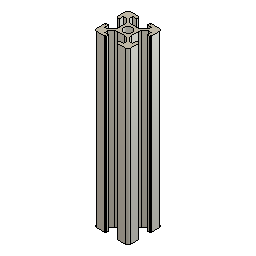
20X20 - T-slot - Aluminium Profile (Autodesk Fusion 360 design; units mm, degrees)
Autodesk Fusion 360 part; units mm, degrees
sketch "Sketch1" plane through (0, 0, 0) normal (0, 1, 0) x (1, 0, 0)
  circle A0 centre (16.6339, -3.4008) radius 2.5
  line L0 (13.0339, 6.0992) -> (13.0339, 6.5992)
  line L1 (6.6339, 0.1992) -> (7.1339, 0.1992)
  line L2 (6.6339, 0.1992) -> (7.1339, 0.1992)
  line L3 (10.0732, 2.0992) -> (8.4339, 2.0992)
  line L4 (11.1339, 4.7992) -> (11.1339, 3.1598)
  line L5 (13.5339, 4.7992) -> (13.5339, 6.0992)
  line L6 (20.2339, 6.5992) -> (20.2339, 6.0992)
  line L7 (19.7339, 6.0992) -> (19.7339, 4.7992)
  line L8 (22.1339, 4.7992) -> (19.7339, 4.7992)
  line L9 (13.5339, 4.7992) -> (11.1339, 4.7992)
  line L10 (20.2339, 6.0992) -> (19.7339, 6.0992)
  line L11 (13.5339, 6.0992) -> (13.0339, 6.0992)
  line L12 (25.1339, 6.5992) -> (20.2339, 6.5992)
  line L13 (13.0339, 6.5992) -> (8.1339, 6.5992)
  line L14 (22.1339, 3.1598) -> (22.1339, 4.7992)
  line L15 (24.8339, 2.0992) -> (23.1945, 2.0992)
  line L16 (26.1339, 0.1992) -> (26.6339, 0.1992)
  line L17 (26.1339, 0.1992) -> (26.6339, 0.1992)
  line L18 (22.1339, 0.1992) -> (22.1339, 0.2882)
  line L19 (24.8339, -0.3008) -> (26.1339, -0.3008)
  line L20 (24.8339, -0.3008) -> (26.1339, -0.3008)
  line L21 (24.8339, -8.9008) -> (24.8339, -6.5008)
  line L22 (24.8339, -0.3008) -> (24.8339, 2.0992)
  line L23 (24.8339, -0.3008) -> (24.8339, 2.0992)
  line L24 (26.1339, -7.0008) -> (26.1339, -6.5008)
  line L25 (26.1339, -0.3008) -> (26.1339, 0.1992)
  line L26 (26.6339, -11.9008) -> (26.6339, -7.0008)
  line L27 (26.6339, 0.1992) -> (26.6339, 5.0992)
  line L28 (20.5339, -5.4117) -> (20.5339, -1.3899)
  line L29 (22.1339, 3.1598) -> (20.059, 1.085)
  line L30 (13.2087, 1.085) -> (11.1339, 3.1598)
  line L31 (12.7339, -1.3899) -> (12.7339, -5.4117)
  line L32 (11.1339, 0.1992) -> (11.2666, 0.1992)
  line L33 (18.6448, 0.4992) -> (14.623, 0.4992)
  line L34 (7.1339, -0.3008) -> (8.4339, -0.3008)
  line L35 (16.6339, -3.4008) -> (14.8661, -1.6331) construction
  line L36 (12.7339, 0.4992) -> (6.6339, 6.5992) construction
  line L37 (6.6339, 6.5992) -> (12.7339, 0.4992) construction
  line L38 (13.5339, -1.3615) -> (13.5339, -1.3216)
  line L39 (21.1197, 0.0243) -> (23.1945, 2.0992)
  line L40 (20.059, -7.8866) -> (22.1339, -9.9615)
  line L41 (14.8661, -1.6331) -> (17.1642, -3.9311) construction
  line L42 (26.6339, 6.5992) -> (16.1035, -3.9311) construction
  line L43 (15.0967, -3.8773) -> (14.9766, -3.9974)
  line L44 (15.854, -3.1201) -> (15.8242, -3.1498)
  line L45 (13.0339, -0.9862) -> (13.0339, -0.8615)
  line L46 (10.0732, 2.0992) -> (12.1481, 0.0243)
  line L47 (20.2339, -4.5168) -> (20.2339, -4.6968)
  line L48 (11.1339, -9.9615) -> (11.1339, -11.6008)
  line L49 (8.4339, 2.0992) -> (8.4339, -0.3008)
  line L50 (8.4339, -6.5008) -> (8.4339, -8.9008)
  line L51 (7.1339, 0.1992) -> (7.1339, -0.3008)
  line L52 (7.1339, -0.3008) -> (8.4339, -0.3008)
  line L53 (8.4339, 2.0992) -> (8.4339, -0.3008)
  line L54 (8.4339, -6.5008) -> (8.4339, -8.9008)
  line L55 (6.6339, 5.0992) -> (6.6339, 0.1992)
  line L56 (6.6339, -7.0008) -> (6.6339, -11.9008)
  line L57 (7.1339, -7.0008) -> (6.6339, -7.0008)
  line L58 (8.4339, -6.5008) -> (7.1339, -6.5008)
  line L59 (8.4339, -6.5008) -> (7.1339, -6.5008)
  line L60 (7.1339, -7.0008) -> (6.6339, -7.0008)
  line L61 (7.1339, -6.5008) -> (7.1339, -7.0008)
  line L62 (12.1481, -6.8259) -> (10.0732, -8.9008)
  line L63 (7.1339, -12.9008) -> (6.6339, -13.4008) construction
  line L64 (11.1339, -11.6008) -> (13.5339, -11.6008)
  line L65 (19.7339, -11.6008) -> (22.1339, -11.6008)
  line L66 (13.0339, -12.9008) -> (13.5339, -12.9008)
  line L67 (19.7339, -12.9008) -> (20.2339, -12.9008)
  line L68 (20.2339, -13.4008) -> (25.1339, -13.4008)
  line L69 (8.4339, -8.9008) -> (10.0732, -8.9008)
  line L70 (13.5339, -12.9008) -> (13.5339, -11.6008)
  line L71 (13.0339, -13.4008) -> (13.0339, -12.9008)
  line L72 (26.1339, -6.5008) -> (24.8339, -6.5008)
  line L73 (26.1339, -6.5008) -> (24.8339, -6.5008)
  line L74 (26.6339, -7.0008) -> (26.1339, -7.0008)
  line L75 (26.6339, -7.0008) -> (26.1339, -7.0008)
  line L76 (24.8339, -8.9008) -> (24.8339, -6.5008)
  line L77 (22.1339, -11.6008) -> (22.1339, -9.9615)
  line L78 (23.1945, -8.9008) -> (24.8339, -8.9008)
  line L79 (23.1945, -8.9008) -> (21.1197, -6.8259)
  line L80 (11.1339, -9.9615) -> (13.2087, -7.8866)
  line L81 (14.8661, -5.1686) -> (13.5339, -6.5008) construction
  line L82 (11.1339, -8.9008) -> (8.4339, -11.6008) construction
  line L83 (19.7339, -11.6008) -> (19.7339, -12.9008)
  line L84 (20.2339, -12.9008) -> (20.2339, -13.4008)
  line L85 (18.4016, -5.1686) -> (19.7339, -6.5008) construction
  line L86 (20.5339, -7.3008) -> (26.6339, -13.4008) construction
  line L87 (14.623, -7.3008) -> (18.6448, -7.3008)
  arc A1 (26.6339, 5.0992) -> (25.1339, 6.5992) centre (25.1339, 5.0992) ccw
  arc A2 (8.1339, 6.5992) -> (6.6339, 5.0992) centre (8.1339, 5.0992) ccw
  arc A3 (6.6339, -11.9008) -> (8.1339, -13.4008) centre (8.1339, -11.9008) ccw
  arc A4 (25.1339, -13.4008) -> (26.6339, -11.9008) centre (25.1339, -11.9008) ccw
  arc A5 (13.2087, 1.085) -> (14.623, 0.4992) centre (14.623, 2.4992) ccw
  arc A6 (18.6448, 0.4992) -> (20.059, 1.085) centre (18.6448, 2.4992) ccw
  arc A7 (21.1197, 0.0243) -> (20.5339, -1.3899) centre (22.5339, -1.3899) ccw
  arc A8 (20.5339, -5.4117) -> (21.1197, -6.8259) centre (22.5339, -5.4117) ccw
  arc A9 (20.059, -7.8866) -> (18.6448, -7.3008) centre (18.6448, -9.3008) ccw
  arc A10 (14.623, -7.3008) -> (13.2087, -7.8866) centre (14.623, -9.3008) ccw
  arc A11 (12.1481, -6.8259) -> (12.7339, -5.4117) centre (10.7339, -5.4117) ccw
  arc A12 (12.7339, -1.3899) -> (12.1481, 0.0243) centre (10.7339, -1.3899) ccw
  line L88 (8.1339, -13.4008) -> (13.0339, -13.4008)
  dimension "d1" = 5
  dimension "d2" = 20
  dimension "d3" = 20
  dimension "d8" = 7.2
  dimension "d10" = 7.2
  dimension "d12" = 7.2
  dimension "d14" = 11
  dimension "d15" = 11
  dimension "d17" = 1.5
  dimension "d18" = 1.5
  dimension "d19" = 2
  measures "d1" diameter of A0
  measures "d8" distance of origin
  measures "d10" distance of origin
  measures "d17" radius of A1
  measures "d18" radius of A2
  measures "d19" radius of A5
extrude "Extrude1" add sketch "Sketch1" along normal blind 100
equation "Length = 100 mm"
